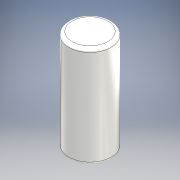
# Autodesk Inventor part: 平行ピン　φ2.5　長さ6
Saved by Autodesk Inventor 2016 (Build 200138000, 138)
## iProperties
Created: 2018-04-05
Part Number: 平行ピン　φ2.5　長さ6
Material: ステンレス鋼
Document SubType Name: Modeling
Designer: Takumi
Density: 8 g/cm^3
Appearance: 半つや出し
Mass: 0.313119 g
Surface Area: 0.712654 cm^2
Volume: 0.0391399 cm^3
Author: Takumi
Autodesk Inventor part; units mm, degrees
ref_plane "YZ Plane" through (0, 0, 0) normal (1, 0, 0) x (0, 1, 0)
ref_plane "XZ Plane" through (0, 0, 0) normal (0, 1, 0) x (-1, 0, 0)
ref_plane "XY Plane" through (0, 0, 0) normal (0, 0, 1) x (1, 0, 0)
sketch "スケッチ1" plane through (0, 0, 0) normal (0, 0, 1) x (1, 0, 0)
  circle A0 centre (0, 0) radius 1.25
  dimension "d0" = 2.5
  constraints: 1 centre point, 1 coincident
  measures "d0" diameter of A0
extrude "押し出し1" add sketch "スケッチ1" along normal blind 6
fillet "フィレット1" radius 0.2 2 edges at (-1.25, 0, 6) (-1.25, 0, 0)
